Autodesk Inventor part; units mm, degrees
(part 2 of 2)
  point P163 (-83.3333, 66.6667)
  point P164 (-91.6667, 66.6667)
  point P165 (-83.3333, 75)
  point P166 (-66.6667, 66.6667)
  point P167 (-75, 66.6667)
  point P168 (-66.6667, 75)
  point P169 (-50, 66.6667)
  point P170 (-58.3333, 66.6667)
  point P171 (-50, 75)
  point P172 (-33.3333, 66.6667)
  point P173 (-41.6667, 66.6667)
  point P174 (-33.3333, 75)
  point P175 (-16.6667, 66.6667)
  point P176 (-25, 66.6667)
  point P177 (-16.6667, 75)
  point P178 (0, 66.6667)
  point P179 (-8.3333, 66.6667)
  point P180 (0, 75)
  point P181 (-83.3333, 83.3333)
  point P182 (-91.6667, 83.3333)
  point P183 (-83.3333, 91.6667)
  point P184 (-66.6667, 83.3333)
  point P185 (-75, 83.3333)
  point P186 (-66.6667, 91.6667)
  point P187 (-50, 83.3333)
  point P188 (-58.3333, 83.3333)
  point P189 (-50, 91.6667)
  point P190 (-33.3333, 83.3333)
  point P191 (-41.6667, 83.3333)
  point P192 (-33.3333, 91.6667)
  point P193 (-16.6667, 83.3333)
  point P194 (-25, 83.3333)
  point P195 (-16.6667, 91.6667)
  point P196 (0, 83.3333)
  point P197 (-8.3333, 83.3333)
  point P198 (0, 91.6667)
  point P199 (16.6667, -83.3333)
  dimension "d108" = 16.6667
  dimension "d109" = 16.6667
  dimension "gridOCell_XOffset" = 91.6667
  dimension "gridOCell_YOffset" = 91.6667
  dimension "d115" = 16.6667
  dimension "d118" = 16.6667
  constraints: 968 end point, 2 collinear, 2 horizontal, 2 midpoint, 2 parallel, 1 horizontal alignment, 1 perpendicular, 1 vertical, 1 vertical alignment, 1318 other
  measures "d108" distance of L84.end L85.end
  measures "d109" distance of L85.end L86.end
  measures "gridOCell_XOffset" horizontal distance of L86.end point (0, 0)
  measures "gridOCell_YOffset" horizontal distance of L86.end point (0, 0)
  measures "d115" distance of L84.start L88.start
  measures "d118" distance of L84.start L108.start
sketch "Sketch24" plane through (0, 0, -18.5) normal (0, 0, 1) x (1, 0, 0)
  line L0 (-88.3333, -80.5833) -> (-78.3333, -80.5833)
  line L1 (-78.3333, -80.5833) -> (-78.3333, -86.0833)
  line L2 (-78.3333, -86.0833) -> (-88.3333, -86.0833)
  line L3 (-88.3333, -86.0833) -> (-88.3333, -80.5833)
  point P0 (0, 0)
  point P1 (-83.3333, -83.3333)
  point P2 (-83.3333, -80.5833)
  point P3 (-88.3333, -83.3333)
  dimension "LEDSlot_height" = 5.5
  dimension "LEDSlot_width" = 10
  constraints: 8 end point, 2 midpoint, 2 parallel, 1 horizontal, 1 horizontal alignment, 1 perpendicular, 1 vertical alignment
  measures "LEDSlot_height" distance of L2.end L0.start
  measures "LEDSlot_width" distance of L1.end L2.end
extrude "Extrusion18" cut sketch "Sketch24" against normal through all bodies 7
sketch "Sketch15" plane through (0, 0, 1.5) normal (0, 0, 1) x (1, 0, 0)
  line L0 (88, 108) -> (108, 108) projected
  line L1 (88, 105) -> (88, 108) projected
  line L2 (88, 105) -> (68.8, 105) projected
  line L3 (68.8, 108) -> (68.8, 105) projected
  line L4 (48.8, 108) -> (68.8, 108) projected
  line L5 (48.8, 105) -> (48.8, 108) projected
  line L6 (48.8, 105) -> (29.6, 105) projected
  line L7 (29.6, 108) -> (29.6, 105) projected
  line L8 (9.6, 108) -> (29.6, 108) projected
  line L9 (9.6, 105) -> (9.6, 108) projected
  line L10 (9.6, 105) -> (-9.6, 105) projected
  line L11 (-9.6, 108) -> (-9.6, 105) projected
  line L12 (-29.6, 108) -> (-9.6, 108) projected
  line L13 (-29.6, 105) -> (-29.6, 108) projected
  line L14 (-29.6, 105) -> (-48.8, 105) projected
  line L15 (-48.8, 108) -> (-48.8, 105) projected
  line L16 (-68.8, 108) -> (-48.8, 108) projected
  line L17 (-68.8, 105) -> (-68.8, 108) projected
  line L18 (-68.8, 105) -> (-88, 105) projected
  line L19 (-88, 108) -> (-88, 105) projected
  line L20 (-108, 108) -> (-88, 108) projected
  line L21 (-108, 108) -> (-108, 88) projected
  line L22 (-108, 88) -> (-105, 88) projected
  line L23 (-105, 88) -> (-105, 68.8) projected
  line L24 (-105, 68.8) -> (-108, 68.8) projected
  line L25 (-108, 68.8) -> (-108, 48.8) projected
  line L26 (-108, 48.8) -> (-105, 48.8) projected
  line L27 (-105, 48.8) -> (-105, 29.6) projected
  line L28 (-105, 29.6) -> (-108, 29.6) projected
  line L29 (-108, 29.6) -> (-108, 9.6) projected
  line L30 (-108, 9.6) -> (-105, 9.6) projected
  line L31 (-105, 9.6) -> (-105, -9.6) projected
  line L32 (-105, -9.6) -> (-108, -9.6) projected
  line L33 (-108, -9.6) -> (-108, -29.6) projected
  line L34 (-108, -29.6) -> (-105, -29.6) projected
  line L35 (-105, -29.6) -> (-105, -48.8) projected
  line L36 (-105, -48.8) -> (-108, -48.8) projected
  line L37 (-108, -48.8) -> (-108, -68.8) projected
  line L38 (-108, -68.8) -> (-105, -68.8) projected
  line L39 (-105, -68.8) -> (-105, -88) projected
  line L40 (-105, -88) -> (-108, -88) projected
  line L41 (-108, -88) -> (-108, -108) projected
  line L42 (-108, -108) -> (-88, -108) projected
  line L43 (-88, -108) -> (-88, -105) projected
  line L44 (-88, -105) -> (-68.8, -105) projected
  line L45 (-68.8, -105) -> (-68.8, -108) projected
  line L46 (-68.8, -108) -> (-48.8, -108) projected
  line L47 (-48.8, -108) -> (-48.8, -105) projected
  line L48 (-48.8, -105) -> (-29.6, -105) projected
  line L49 (-29.6, -105) -> (-29.6, -108) projected
  line L50 (-29.6, -108) -> (-9.6, -108) projected
  line L51 (-9.6, -108) -> (-9.6, -105) projected
  line L52 (-9.6, -105) -> (9.6, -105) projected
  line L53 (9.6, -105) -> (9.6, -108) projected
  line L54 (9.6, -108) -> (29.6, -108) projected
  line L55 (29.6, -108) -> (29.6, -105) projected
  line L56 (29.6, -105) -> (48.8, -105) projected
  line L57 (48.8, -105) -> (48.8, -108) projected
  line L58 (48.8, -108) -> (68.8, -108) projected
  line L59 (68.8, -108) -> (68.8, -105) projected
  line L60 (68.8, -105) -> (88, -105) projected
  line L61 (88, -105) -> (88, -108) projected
  line L62 (88, -108) -> (108, -108) projected
  line L63 (108, -108) -> (108, -88) projected
  line L64 (105, -88) -> (108, -88) projected
  line L65 (105, -88) -> (105, -68.8) projected
  line L66 (108, -68.8) -> (105, -68.8) projected
  line L67 (108, -48.8) -> (108, -68.8) projected
  line L68 (105, -48.8) -> (108, -48.8) projected
  line L69 (105, -48.8) -> (105, -29.6) projected
  line L70 (108, -29.6) -> (105, -29.6) projected
  line L71 (108, -9.6) -> (108, -29.6) projected
  line L72 (105, -9.6) -> (108, -9.6) projected
  line L73 (105, -9.6) -> (105, 9.6) projected
  line L74 (108, 9.6) -> (105, 9.6) projected
  line L75 (108, 29.6) -> (108, 9.6) projected
  line L76 (105, 29.6) -> (108, 29.6) projected
  line L77 (105, 29.6) -> (105, 48.8) projected
  line L78 (108, 48.8) -> (105, 48.8) projected
  line L79 (108, 68.8) -> (108, 48.8) projected
  line L80 (105, 68.8) -> (108, 68.8) projected
  line L81 (105, 68.8) -> (105, 88) projected
  line L82 (108, 88) -> (105, 88) projected
  line L83 (108, 108) -> (108, 88) projected
  line L84 (-89, 109) -> (-89, 106)
  line L85 (-89, 106) -> (-69.8, 106)
  line L86 (-69.8, 106) -> (-69.8, 109)
  line L87 (-69.8, 109) -> (-49.8, 109)
  line L88 (-49.8, 109) -> (-49.8, 106)
  line L89 (-49.8, 106) -> (-30.6, 106)
  line L90 (-30.6, 106) -> (-30.6, 109)
  line L91 (-30.6, 109) -> (-10.6, 109)
  line L92 (-10.6, 109) -> (-10.6, 106)
  line L93 (-10.6, 106) -> (10.6, 106)
  line L94 (10.6, 106) -> (10.6, 109)
  line L95 (10.6, 109) -> (30.6, 109)
  line L96 (30.6, 109) -> (30.6, 106)
  line L97 (30.6, 106) -> (49.8, 106)
  line L98 (49.8, 106) -> (49.8, 109)
  line L99 (49.8, 109) -> (69.8, 109)
  line L100 (69.8, 109) -> (69.8, 106)
  line L101 (69.8, 106) -> (89, 106)
  line L102 (89, 106) -> (89, 109)
  line L103 (89, 109) -> (109, 109)
  line L104 (109, 109) -> (109, 89)
  line L105 (109, 89) -> (106, 89)
  line L106 (106, 89) -> (106, 69.8)
  line L107 (106, 69.8) -> (109, 69.8)
  line L108 (109, 69.8) -> (109, 49.8)
  line L109 (109, 49.8) -> (106, 49.8)
  line L110 (106, 49.8) -> (106, 30.6)
  line L111 (106, 30.6) -> (109, 30.6)
  line L112 (109, 30.6) -> (109, 10.6)
  line L113 (109, 10.6) -> (106, 10.6)
  line L114 (106, 10.6) -> (106, -10.6)
  line L115 (106, -10.6) -> (109, -10.6)
  line L116 (109, -10.6) -> (109, -30.6)
  line L117 (109, -30.6) -> (106, -30.6)
  line L118 (106, -30.6) -> (106, -49.8)
  line L119 (106, -49.8) -> (109, -49.8)
  line L120 (109, -49.8) -> (109, -69.8)
  line L121 (109, -69.8) -> (106, -69.8)
  line L122 (106, -69.8) -> (106, -89)
  line L123 (106, -89) -> (109, -89)
  line L124 (109, -89) -> (109, -109)
  line L125 (109, -109) -> (89, -109)
  line L126 (89, -109) -> (89, -106)
  line L127 (89, -106) -> (69.8, -106)
  line L128 (69.8, -106) -> (69.8, -109)
  line L129 (69.8, -109) -> (49.8, -109)
  line L130 (49.8, -109) -> (49.8, -106)
  line L131 (49.8, -106) -> (30.6, -106)
  line L132 (30.6, -106) -> (30.6, -109)
  line L133 (30.6, -109) -> (10.6, -109)
  line L134 (10.6, -109) -> (10.6, -106)
  line L135 (10.6, -106) -> (-10.6, -106)
  line L136 (-10.6, -106) -> (-10.6, -109)
  line L137 (-10.6, -109) -> (-30.6, -109)
  line L138 (-30.6, -109) -> (-30.6, -106)
  line L139 (-30.6, -106) -> (-49.8, -106)
  line L140 (-49.8, -106) -> (-49.8, -109)
  line L141 (-49.8, -109) -> (-69.8, -109)
  line L142 (-69.8, -109) -> (-69.8, -106)
  line L143 (-69.8, -106) -> (-89, -106)
  line L144 (-89, -106) -> (-89, -109)
  line L145 (-89, -109) -> (-109, -109)
  line L146 (-109, -109) -> (-109, -89)
  line L147 (-109, -89) -> (-106, -89)
  line L148 (-106, -89) -> (-106, -69.8)
  line L149 (-106, -69.8) -> (-109, -69.8)
  line L150 (-109, -69.8) -> (-109, -49.8)
  line L151 (-109, -49.8) -> (-106, -49.8)
  line L152 (-106, -49.8) -> (-106, -30.6)
  line L153 (-106, -30.6) -> (-109, -30.6)
  line L154 (-109, -30.6) -> (-109, -10.6)
  line L155 (-109, -10.6) -> (-106, -10.6)
  line L156 (-106, -10.6) -> (-106, 10.6)
  line L157 (-106, 10.6) -> (-109, 10.6)
  line L158 (-109, 10.6) -> (-109, 30.6)
  line L159 (-109, 30.6) -> (-106, 30.6)
  line L160 (-106, 30.6) -> (-106, 49.8)
  line L161 (-106, 49.8) -> (-109, 49.8)
  line L162 (-109, 49.8) -> (-109, 69.8)
  line L163 (-109, 69.8) -> (-106, 69.8)
  line L164 (-106, 69.8) -> (-106, 89)
  line L165 (-106, 89) -> (-109, 89)
  line L166 (-109, 89) -> (-109, 109)
  line L167 (-109, 109) -> (-89, 109)
  point P0 (0, 0)
  dimension "d70" = 1
  constraints: 168 end point, 83 other
  measures "d70" distance between parallel lines of L20 L167
pattern_linear "LEDSlots" count 11 spacing 16.6667 along (1, 0, 0) count 11 spacing 16.6667 along (0, 1, 0) of "Extrusion18" bodies 7
sketch "Sketch25" plane through (0, 0, -18.5) normal (0, 0, 1) x (1, 0, 0)
  line L0 (-93.1667, 105) -> (-90.1667, 105)
  line L1 (-90.1667, 105) -> (-90.1667, -105)
  line L2 (-90.1667, -105) -> (-93.1667, -105)
  line L3 (-93.1667, -105) -> (-93.1667, 105)
  line L4 (-91.6667, -91.6667) -> (-91.6667, -75) construction
  line L5 (-75, -91.6667) -> (-91.6667, -91.6667) construction
  point P0 (0, 0)
  point P1 (-90.1667, 0)
  point P2 (-91.6667, -105)
  dimension "GridThickness" = 3
  dimension "d132" = 210
  constraints: 8 end point, 2 midpoint, 2 parallel, 1 horizontal, 1 horizontal alignment, 1 perpendicular, 1 vertical alignment
  measures "GridThickness" distance of L0.start L0.end
  measures "d132" distance of L2.end L0.start
extrude "GridVertMasterBase" add sketch "Sketch25" along normal blind 17 separate body
sketch "GridVertTabMaster" plane through (0, 0, -18.5) normal (0, 0, -1) x (-1, 0, 0)
  line L0 (90.1667, 105) -> (90.1667, -105) projected
  line L1 (93.1667, -105) -> (93.1667, 105) projected
  line L2 (93.1667, -89.1667) -> (90.1667, -89.1667)
  line L3 (90.1667, -89.1667) -> (90.1667, -94.1667)
  line L4 (90.1667, -94.1667) -> (93.1667, -94.1667)
  line L5 (93.1667, -94.1667) -> (93.1667, -89.1667)
  point P0 (0, 0)
  point P1 (90.1667, -91.6667)
  point P2 (90.1667, 0)
  point P3 (93.1667, -91.6667)
  point P4 (93.1667, 0)
  dimension "d151" = 5
  dimension "d152" = 91.6667
  constraints: 8 end point, 4 midpoint, 2 parallel, 2 vertical alignment, 1 horizontal, 1 perpendicular
  measures "d151" distance of L4.end L2.start
  measures "d152" vertical distance of point (0, 0) point (90.167, -91.667)
sketch "GridVertSlotMaster" plane through (0, 0, -18.5) normal (0, 0, -1) x (-1, 0, 0)
  line L0 (90.1667, 105) -> (90.1667, -105) projected
  line L1 (93.1667, -105) -> (93.1667, 105) projected
  line L2 (90.1667, -89.1667) -> (93.1667, -89.1667)
  line L3 (93.1667, -89.1667) -> (93.1667, -94.1667)
  line L4 (93.1667, -94.1667) -> (90.1667, -94.1667)
  line L5 (90.1667, -94.1667) -> (90.1667, -89.1667)
  line L6 (93.1667, -89.1667) -> (90.1667, -89.1667) projected
  line L7 (90.1667, -94.1667) -> (93.1667, -94.1667) projected
  point P0 (0, 0)
  point P1 (91.6667, -89.1667)
  point P2 (91.6667, -89.1667)
  point P3 (91.6667, -94.1667)
  point P4 (91.6667, -94.1667)
  point P5 (93.1667, -91.6667)
  point P6 (93.1667, 0)
  point P7 (90.1667, -91.6667)
  point P8 (90.1667, 0)
  constraints: 8 end point, 8 midpoint, 2 coincident, 2 parallel, 2 vertical alignment, 1 horizontal, 1 perpendicular
extrude "GridVertTab" add sketch "GridVertTabMaster" along normal blind 3 bodies 8
pattern_linear "GridVertTabs" count 12 spacing 16.6667 along (0, 1, 0) of "GridVertTab" bodies 8
extrude "Extrusion23" cut sketch "GridVertSlotMaster" along normal through all both and the other way through all bodies 7
pattern_linear "GridVertSlotsMaster" count 12 spacing 16.6667 along (0, 1, 0) of "Extrusion23" bodies 7
pattern_linear "GridVertSlots" count 12 spacing 16.6667 along (1, 0, 0) of "Extrusion23", "GridVertSlotsMaster" bodies 7
ref_plane "Work Plane3" through (0, 0, 0) normal (0, 1, 0) x (-1, 0, 0)
equation "\"FrontFaceBaseWidth\" = ClockWidth - 2 * FrontFaceTabDepth"
equation "\"FrontFaceBaseHeight\" = ClockHeight - 2 * FrontFaceTabDepth"
equation "\"FrontFaceThickness\" = Ply3mm"
equation "\"d6\" = TabDepth"
equation "\"FrontFaceTabWidth\" = TabWidth"
equation "\"d8\" = FrontFaceTabDepth"
equation "\"d9\" = FrontFaceThickness"
equation "\"d14\" = FrontFaceTabDepth"
equation "\"d15\" = FrontFaceTabDepth"
equation "\"d16\" = FrontFaceTabWidth"
equation "\"d17\" = FrontFaceThickness"
equation "\"d68\" = ClockWidth"
equation "\"d69\" = ClockDepth"
equation "\"TopFaceThickness\" = Ply3mm"
equation "\"d25\" = FrontFaceTabWidth"
equation "\"TopFaceFrontSlotDepth\" = FrontFaceThickness"
equation "\"d27\" = TopFaceThickness"
equation "\"d33\" = TabDepth"
equation "\"d34\" = TopFaceThickness"
equation "\"d38\" = FrontFaceTopTabSpacing"
equation "\"SideFaceBaseHeight\" = ClockHeight - 2 * FrontFaceThickness"
equation "\"SideFaceBaseDepth\" = ClockDepth"
equation "\"SideFaceThickness\" = Ply3mm"
equation "\"SideFaceTabWidth\" = TopSideSlotWidth"
equation "\"SideTopTabDepth\" = TopFaceThickness"
equation "\"d56\" = SideFaceThickness"
equation "\"d60\" = TopFaceSlotsSideSpcaing"
equation "\"d61\" = FrontFaceThickness"
equation "\"d62\" = FrontFaceTabWidth"
equation "\"d63\" = SideFaceThickness"
equation "\"d67\" = FrontFaceSideTabSpacing"
equation "\"d76\" = FrontFaceBaseHeight"
equation "\"d77\" = FrontFaceBaseWidth"
equation "\"MiddleThickness\" = Ply3mm"
equation "\"d80\" = SideFaceThickness"
equation "\"MiddleTabWidth\" = TabWidth"
equation "\"d82\" = Ply3mm"
equation "\"d86\" = MiddleSideTabSpacing"
equation "\"d87\" = TopFaceThickness"
equation "\"MiddleBottomTabWidth\" = MiddleTabWidth"
equation "\"d89\" = MiddleThickness"
equation "\"d93\" = MiddleBottomTabSpacing"
equation "\"d94\" = TopFaceThickness"
equation "\"d95\" = MiddleBottomTabWidth"
equation "\"d96\" = MiddleThickness"
equation "\"d100\" = MiddleBottomTabSpacing"
equation "\"d101\" = SideFaceThickness"
equation "\"d102\" = MiddleTabWidth"
equation "\"d103\" = MiddleThickness"
equation "\"d70\" = kerf"
equation "\"FrontFaceTabDepth\" = TabDepth"
equation "\"ClockHeight\" = 216"
equation "\"ClockWidth\" = 216"
equation "\"ClockDepth\" = 60"
equation "\"Ply3mm\" = 3"
equation "\"TabDepth\" = Ply3mm"
equation "\"TabWidth\" = 20"
equation "\"kerf\" = 1"
equation "\"MiddleFrontSeparation\" = 17"
equation "\"MiddleSideTabSpacing\" = 2 * MiddleTabWidth"
equation "\"MiddleBottomTabSpacing\" = MiddleSideTabSpacing"
equation "\"gridCellHeight\" = 16.66667"
equation "\"gridCellWidth\" = 16.66667"
equation "\"gridVertTabWidth\" = 5"
equation "\"FrontFaceTopTabSpacing\" = 39.2"
equation "\"TopFaceSlotsSideSpcaing\" = 40"
equation "\"FrontFaceSideTabSpacing\" = 39.2"
